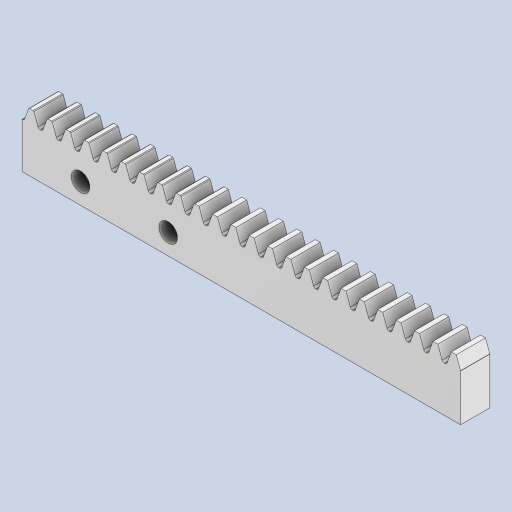
# Autodesk Inventor part: rackgear
Saved by Autodesk Inventor 2023 (Build 270158000, 158)
## iProperties
Category: PARTsolutions
Company: MISUMI
Created: 2024-11-28
Part Number: rackgear
Material: ABS プラスチック
Catalog Web Link: www.cadenas.de
Description: RGEAL, RGEABL, RGEASL, RGEAML-Rack Gears L Dimension Configurable (One End Machined) - Pressure Angle 20 - Hole Position Configurable
Vendor: MISUMI
Document SubType Name: Modeling
Designer: psAdmin
Manufacturer: MISUMI
Mass: 2.6861 g
Surface Area: 16.0116 cm^2
Volume: 2.6861 cm^3
Density: 1.06 g/cm^3
Appearance: 滑らか - 白
PSOL_IDENT_0: {$CADENAS_DATA/23d-libs/misumi/metric/54_spur_gears/rgeasl.prj},239 {VTYP=3D},{NB=RGEASL1.0N-30},{LI
PSOL_IDENT_1: NA=RGEASL1.0N-30},{NN=RGEAL, RGEABL, RGEASL, RGEAML},{DATE=29.05.2023 09:31:20},{GEOMDATE=18.01.2021
PSOL_IDENT_2: 08:14:07},{VERSION=},{LINEID=30},{WBVAR=MAT,HM,L,A,B,C,D,ALT1,ALT2,MS,ALT3,TPC},{WBNUMERIC=L,A,B,C,
PSOL_IDENT_3: D,MS}  {NB=RGEASL1.0N-30},{LINA=RGEASL1.0N-30},{KT=DUMMY},{PN=RGEASL1.0N-30},{MAT=3},{MATALG='1','Fr
PSOL_IDENT_4: ee-Cutting Brass Bar','2','1045 Carbon Steel Equivalent','3','304 Stainless Steel','4','MC Nylon', '
PSOL_IDENT_5: 5','Polyacetal' },{TYPE=RGEASL},{MOD=1.0},{MOD1=1.0},{HM=N},{HMALG='N','No Hole Machining','HT','Bac
PSOL_IDENT_6: k Tapped','ST','Side Tapped','Z','Side Counterbore'},{L=30},{LALG=[20:980/1]},{DD21=6.5},{M12=3},{M1=
PSOL_IDENT_7: 0},{A=0},{AALG=0},{AMIN=0},{AMAX=25},{B=0},{BALG=0},{BMIN=0},{BMAX=25},{C=0},{CALG=0},{CMIN=0},{CMAX=
PSOL_IDENT_8: 25},{D=0},{DALG=0},{DMIN=0},{DMAX=25},{PITCH=3.142},{W=10},{H=10},{HH=9.0},{DD1=3.5},{DD2=6.5},{Z1=3
PSOL_IDENT_9: .5},{M=-},{ALT1= },{ALT1ALG= ' ', 'w/o MC (One End Female Thread Machining)', 'MC', 'with MC (One En
PSOL_IDENT_10: d Female Thread Machining)' },{ALT2= },{ALT2ALG= ' ', 'w/o WMC (Both Ends Female Thread Machining)',
PSOL_IDENT_11: 'WMC', 'with WMC (Both Ends Female Thread Machining)' },{ALT2ALGMAX=30},{MS=0},{MSALG=0},{ALT3=},{A
PSOL_IDENT_12: LT3ALG= '','Not applicable' },{TPC=N/A},{TPCA= 'N/A' },{APN=},{BPN=},{CPN=},{DPN=},{MCPN=},{WMCPN=},
PSOL_IDENT_13: {MSPN=},{ALT3PN=},{TED=2.250},{SP=1.571},{PFP=0.38},{HAP=1},{HFP=1.25},{DEG1=20},{NN=9},{L3=1.14947}
PSOL_IDENT_14: ,{NN1=10},{MC3DL1=0.000},{MC3DL2=0.000},{MCCIF3D=2.000}
NB: RGEASL1.0N-30
NN: RGEAL, RGEABL, RGEASL, RGEAML
NT: Rack Gears L Dimension Configurable (One End Machined) - Pressure Angle 20 - Hole Position Configurable
NBSYN: $PN.
LINA: RGEASL1.0N-30
CATALOG: Misumi
PN: RGEASL1.0N-30
MAT: 304 Stainless Steel
MOD: 1.0
HM: No Hole Machining
L: 30
A: 0
B: 0
C: 0
D: 0
PITCH: 3.142
W: 10
H: 10
HH: 9
DD1: 3.5
DD2: 6.5
Z1: 3.5
M: -
ALT1: w/o MC (One End Female Thread Machining)
ALT2: w/o WMC (Both Ends Female Thread Machining)
MS: 0
ALT3: Not applicable
TPC: N/A
SUPPLIER: MISUMI
ARTICLENO: RGEASL1.0N-30
BOMINFO: RGEASL1.0N-30
CREATOR: CADENAS GmbH
Title: RGEASL1.0N-30
Author: Cadenas PARTsolutions
Comments: Rack Gears L Dimension Configurable (One End Machined) - Pressure Angle 20 - Hole Position Configurable
Autodesk Inventor part; units mm, degrees
ref_plane "YZ Plane" through (0, 0, 0) normal (1, 0, 0) x (0, 1, 0)
ref_plane "XZ Plane" through (0, 0, 0) normal (0, 1, 0) x (-1, 0, 0)
ref_plane "XY Plane" through (0, 0, 0) normal (0, 0, 1) x (1, 0, 0)
sketch "Sketch_1" plane through (0, 0, 0) normal (0, 0, 1) x (1, 0, 0)
  line L0 (0, 10) -> (0, 0)
  line L1 (0, 0) -> (75, 0)
  line L2 (75, 0) -> (75, 10)
  line L3 (75, 10) -> (0, 10)
  dimension "d13" = 10
  dimension "d14" = 75
  constraints: 8 end point, 2 horizontal, 2 vertical
  measures "d13" distance of L0.start L0.end
  measures "d14" distance of L2.end L0.start
extrude "Extrusion1" add sketch "Sketch_1" along normal blind 5
sketch "_____14" plane through (0, 0, 0) normal (0, 0, 1) x (1, 0, 0)
  line L0 (-1.1495, 10) -> (-0.4215, 8)
  arc A0 (-0.4215, 8) -> (-0.0645, 7.75) centre (-0.0645, 8.13) ccw
  line L1 (-0.0645, 7.75) -> (0.0645, 7.75)
  arc A1 (0.0645, 7.75) -> (0.4215, 8) centre (0.0645, 8.13) ccw
  line L2 (0.4215, 8) -> (1.1495, 10)
  line L3 (1.1495, 10) -> (-1.1495, 10)
  constraints: 8 end point, 4 point on circle, 2 centre point
extrude "Extrusion2" cut sketch "_____14" along normal blind 10
pattern_linear "Rectangular Pattern1" count 30 spacing 3.142 along (1, 0, 0) of "Extrusion2"
chamfer "面取り1" distance 0.1 angle 45 19 edges at (1.1495, 10, 2.5) (1.9925, 10, 2.5) (4.2915, 10, 2.5) (5.1345, 10, 2.5) (7.4335, 10, 2.5) (8.2765, 10, 2.5) (10.5755, 10, 2.5) (11.4185, 10, 2.5) (13.7175, 10, 2.5) (14.5605, 10, 2.5) (17.7025, 10, 2.5) (16.8595, 10, 2.5) (20.0015, 10, 2.5) (20.8445, 10, 2.5) (23.1435, 10, 2.5) (23.9865, 10, 2.5) (26.2855, 10, 2.5) (27.1285, 10, 2.5) (29.4275, 10, 2.5)
sketch "スケッチ4" plane through (0, 0, 0) normal (0, 0, -1) x (-1, 0, 0)
  circle A0 centre (-25, 3.5) radius 2.85
  circle A1 centre (-10, 3.5) radius 2.85
  circle A2 centre (-10, 3.5) radius 1.6
  circle A3 centre (-25, 3.5) radius 1.6
  line L0 (0, 0) -> (-75, 0) projected
  line L1 (0, 7.75) -> (0, 0) projected
  dimension "d23" = 3.2
  dimension "d24" = 5.7
  dimension "d25" = 3.2
  dimension "d26" = 5.7
  dimension "d29" = 15
  dimension "d30" = 3.5
  dimension "d31" = 3.5
  dimension "d32" = 10
  constraints: 4 centre point, 2 coincident
  measures "d23" diameter of A3
  measures "d24" diameter of A0
  measures "d25" diameter of A2
  measures "d26" diameter of A1
  measures "d29" distance of A1.centre A0.centre
  measures "d30" distance from line of L0 A1.centre
  measures "d31" distance from line of L0 A0.centre
  measures "d32" distance from line of L1 A1.centre
extrude "押し出し3" cut sketch "スケッチ4" against normal blind 5 contours A2 | A3
extrude "押し出し4" cut sketch "スケッチ4" against normal blind 3 contours A0 | A1 | A2 | A3
body "Solid1"
